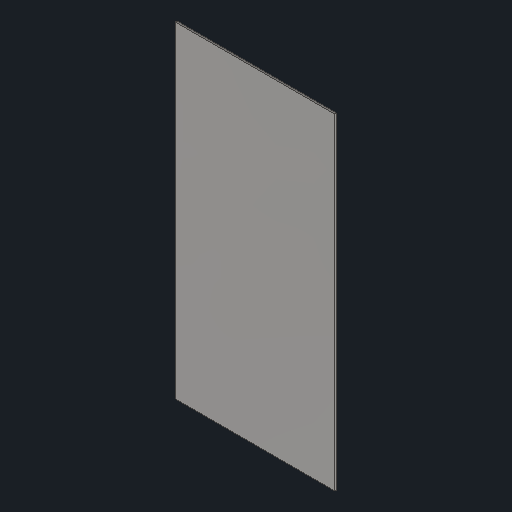
# Autodesk Inventor part: SuperStructure
Saved by Autodesk Inventor 2024 (Build 280153000, 153)
## iProperties
Created: 2025-02-08
Part Number: SuperStructure
Material: Stainless Steel
Document SubType Name: Sheet Metal
Designer: Tommy Rohmann
Density: 8 g/cm^3
Sheet Metal Rule: Default
Appearance: Semi-Polished
Author: Tommy Rohmann
Autodesk Inventor part; units mm, degrees
ref_plane "YZ Plane" through (0, 0, 0) normal (1, 0, 0) x (0, 1, 0)
ref_plane "XZ Plane" through (0, 0, 0) normal (0, 1, 0) x (-1, 0, 0)
ref_plane "XY Plane" through (0, 0, 0) normal (0, 0, 1) x (1, 0, 0)
sketch "SuperStructure" plane through (0, 0, 0) normal (0, 0, 1) x (1, 0, 0)
  line L0 (-519.3392, 0) -> (-735.2392, 0)
  line L1 (-786.0392, 0) -> (-786.0392, 544.83)
  line L2 (-786.0392, 544.83) -> (-735.2392, 544.83)
  line L3 (-519.3392, 544.83) -> (-519.3392, 0)
  line L4 (-735.2392, 544.83) -> (-735.2392, 0)
  line L5 (-735.2392, 544.83) -> (-519.3392, 544.83)
  line L6 (-735.2392, 0) -> (-786.0392, 0)
  point P0 (-680.2058, 272.415)
  dimension "d448" = 266.7
  dimension "d449" = 544.83
  dimension "d451" = 215.9
  measures "d448" distance of L1.end L3.start
  measures "d449" distance of L1.start L1.end
  measures "d451" distance between parallel lines of L3 L4
derived "LAYOUT.ipt"
sketch "Sketch1" plane through (0, 0, 0) normal (0, 0, 1) x (1, 0, 0)
  line L0 (-519.3392, 0) -> (-735.2392, 0)
  line L1 (-786.0392, 0) -> (-786.0392, 544.83)
  line L2 (-786.0392, 544.83) -> (-735.2392, 544.83)
  line L3 (-519.3392, 544.83) -> (-519.3392, 0)
  line L4 (-735.2392, 544.83) -> (-735.2392, 0)
  line L5 (-735.2392, 544.83) -> (-519.3392, 544.83)
  line L6 (-735.2392, 0) -> (-786.0392, 0)
extrude "Plate2" add sketch "Sketch1" along normal blind 3.048
equation "\"d2\" = Thickness"
equation "\"BendRadius\" = Thickness"
equation "\"BendReliefWidth\" = Thickness"
equation "\"BendReliefDepth\" = 0.5 * Thickness"
equation "\"CornerReliefSize\" = 4 * Thickness"
equation "\"MinimumRemnant\" = 2 * Thickness"
equation "\"TransitionRadius\" = BendRadius"
equation "\"JacobiRadiusSize\" = BendRadius"
equation "\"GapSize\" = Thickness"
equation "\"Thickness\" = 3.048"
body "Solid2"
